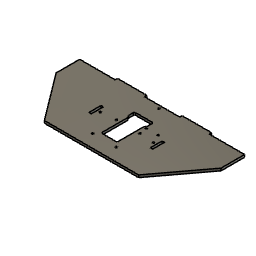
tablet_bottom_plate (Autodesk Fusion 360 design; units mm, degrees)
Autodesk Fusion 360 part; units mm, degrees
note: some values were not read from the file. Set by a fixed rule: the direction of a hole.
sketch "スケッチ1" plane through (0, 0, 0) normal (0, 1, 0) x (1, 0, 0)
  line L0 (140, -4) -> (140, -44)
  line L1 (140, -44) -> (80, -124)
  line L2 (80, -124) -> (-80, -124)
  line L3 (-80, -124) -> (-140, -44)
  line L4 (-140, -44) -> (-140, -4)
  line L5 (50, -54) -> (54, -54)
  line L6 (54, -54) -> (54, -74)
  line L7 (54, -74) -> (50, -74)
  line L8 (50, -74) -> (50, -54)
  line L9 (-54, -54) -> (-50, -54)
  line L10 (-50, -54) -> (-50, -74)
  line L11 (-50, -74) -> (-54, -74)
  line L12 (-54, -74) -> (-54, -54)
  line L13 (50, -64) -> (45, -64)
  line L14 (-50, -64) -> (-45, -64)
  line L15 (-140, -4) -> (-80, -4)
  line L16 (-80, -4) -> (-80, 0)
  line L17 (-80, 0) -> (-30, 0)
  line L18 (-30, 0) -> (-30, -4)
  line L19 (-30, -4) -> (30, -4)
  line L20 (30, -4) -> (30, 0)
  line L21 (30, 0) -> (80, 0)
  line L22 (80, 0) -> (80, -4)
  line L23 (80, -4) -> (140, -4)
  line L24 (0, -4) -> (0, -9)
  line L25 (-10, -96) -> (10, -96)
  line L26 (10, -96) -> (10, -92)
  line L27 (10, -92) -> (-10, -92)
  line L28 (-10, -92) -> (-10, -96)
  line L29 (-60, -78.5) -> (60, -78.5)
  line L30 (-75, -96) -> (-55, -96)
  line L31 (-55, -96) -> (-55, -104)
  line L32 (-55, -104) -> (-75, -104)
  line L33 (-75, -104) -> (-75, -96)
  line L34 (-20, -62) -> (20, -62)
  line L35 (20, -62) -> (20, -102)
  line L36 (20, -102) -> (-20, -102)
  line L37 (-20, -102) -> (-20, -62)
  line L38 (-13.5, -47) -> (13.5, -47)
  line L39 (13.5, -47) -> (13.5, -94)
  line L40 (13.5, -94) -> (-13.5, -94)
  line L41 (-13.5, -94) -> (-13.5, -47)
  line L42 (-16, -35) -> (16, -35)
  line L43 (16, -35) -> (16, -47)
  line L44 (16, -47) -> (-16, -47)
  line L45 (-16, -47) -> (-16, -35)
  point P0 (0, -124)
  point P1 (0, -4)
  point P2 (0, -96)
  point P3 (0, -78.5)
  point P4 (0, -62)
  point P5 (0, -47)
  dimension "d1" = 280
  dimension "d2" = 40
  dimension "d3" = 80
  dimension "d4" = 160
  dimension "d8" = 20
  dimension "d9" = 4
  dimension "d10" = 50
  dimension "d11" = 50
  dimension "d12" = 5
  dimension "d13" = 5
  dimension "d17" = 4
  dimension "d18" = 60
  dimension "d19" = 60
  dimension "d20" = 60
  dimension "d22" = 50
  dimension "d23" = 5
  dimension "d24" = 28
  dimension "d25" = 4
  dimension "d26" = 20
  dimension "d27" = 13.5
  dimension "d28" = 120
  dimension "d29" = 20
  dimension "d30" = 8
  dimension "d31" = 45
  dimension "d32" = 40
  dimension "d33" = 40
  dimension "d34" = 62
  dimension "d35" = 27
  dimension "d36" = 15
  dimension "d37" = 32
  dimension "d38" = 12
  dimension "d39" = 32
  constraint vertical L4
  constraint equal L1 L3
  constraint equal L0 L4
  constraint horizontal L5
  constraint vertical L6
  constraint horizontal L7
  constraint vertical L8
  constraint horizontal L9
  constraint vertical L10
  constraint horizontal L11
  constraint vertical L12
  constraint collinear L5 L9
  constraint collinear L7 L11
  constraint equal L5 L9
  constraint midpoint L8 L13.start
  constraint perpendicular L8 L13
  constraint midpoint L10 L14.start
  constraint perpendicular L10 L14
  constraint horizontal L2
  constraint vertical L0
  constraint horizontal L0.end L3.end
  constraint perpendicular L4 L15
  constraint perpendicular L15 L16
  constraint perpendicular L16 L17
  constraint perpendicular L15 L18
  constraint perpendicular L18 L19
  constraint perpendicular L19 L20
  constraint perpendicular L20 L21
  constraint perpendicular L19 L22
  constraint perpendicular L22 L23
  constraint coincident L0.start L23.end
  constraint midpoint L2 P0
  constraint midpoint L19 P1
  constraint vertical origin P1
  constraint vertical P0 P1
  constraint collinear L19 L23
  constraint collinear L17 L21
  constraint horizontal origin L20.end
  constraint coincident P1 L24.start
  constraint perpendicular L19 L24
  constraint horizontal L25
  constraint vertical L26
  constraint horizontal L27
  constraint vertical L28
  constraint midpoint L25 P2
  constraint vertical P0 P2
  constraint parallel L27 L29
  constraint midpoint L29 P3
  constraint vertical P0 P3
  constraint horizontal L30
  constraint vertical L31
  constraint horizontal L32
  constraint vertical L33
  constraint collinear L25 L30
  constraint horizontal L34
  constraint vertical L35
  constraint horizontal L36
  constraint vertical L37
  constraint midpoint L34 P4
  constraint vertical origin P4
  constraint horizontal L38
  constraint vertical L39
  constraint horizontal L40
  constraint vertical L41
  constraint midpoint L38 P5
  constraint vertical origin P5
  constraint horizontal L42
  constraint vertical L43
  constraint horizontal L44
  constraint vertical L45
  constraint midpoint P5 L44
  measures "d1" distance of L0.start L4.end
  measures "d2" distance of L0.start L0.end
  measures "d3" vertical distance of L0.end L1.end
  measures "d4" distance of L1.end L2.end
  measures "d8" distance of L5.end L6.end
  measures "d9" distance of L6.end L7.end
  measures "d10" distance of origin L8
  measures "d11" distance of origin L10
  measures "d12" distance of L14.start L14.end
  measures "d13" distance of L13.start L13.end
  measures "d17" distance of L15.end L16.end
  measures "d18" distance of L18.end L19.end
  measures "d19" distance of L4.end L15.end
  measures "d20" distance of L22.end L0.start
  measures "d22" distance of L5 L19
  measures "d23" distance of P1 L24.end
  measures "d24" distance of L2 L25
  measures "d25" distance of L25.end L26.end
  measures "d26" distance of L26.end L27.end
  measures "d27" distance of L27 L29
  measures "d28" distance of L29.start L29.end
  measures "d29" distance of L30.start L30.end
  measures "d30" distance of L30.start L32.end
  measures "d31" distance of L25.start L31
  measures "d32" distance of L34.start L34.end
  measures "d33" distance of L34.end L35.end
  measures "d34" distance of origin L34
  measures "d35" distance of L38.start L38.end
  measures "d36" distance of L34 L38
  measures "d37" distance of L34 L40
  measures "d38" distance of L42 L44
  measures "d39" distance of L42.start L42.end
extrude "押し出し1" add sketch "スケッチ1" along normal blind 4 contours L0 L1 L2 L3 L4 L15 L16 L17 L18 L19 L20 L21 L22 L23 | L25 L26 L28 L40 | L25 L26 L28 L29 L35 L36 L37 L39 L40 L41 | L29 L34 L37 L41 | L29 L34 L35 L39 | L30 L31 L32 L33
hole "穴1" at (-45, 0, 64) at (45, 0, 64) at (0, 0, 9) at (-20, 0, 102) at (-20, 0, 62) at (20, 0, 62) at (20, 0, 102) direction (0, 1, 0) diameter 3.2 depth 4 tip angle 118
fillet "フィレット1" radius 2 8 edges at (-16, 2, 35) (16, 2, 35) (16, 2, 47) (13.5, 2, 47) (-16, 2, 47) (-13.5, 2, 47) (-13.5, 2, 94) (13.5, 2, 94)
sketch "スケッチ2" plane through (0, 4, 0) normal (0, 1, 0) x (-1, 0, 0)
  circle A0 centre (-20, 62) radius 1.6
  circle A1 centre (20, 102) radius 1.6
  circle A2 centre (-45, 64) radius 1.6
  circle A3 centre (45, 64) radius 1.6
  circle A4 centre (0, 9) radius 1.6
  circle A5 centre (20, 62) radius 1.6
  circle A6 centre (-20, 102) radius 1.6
  line L0 (-54, 74) -> (-50, 74)
  line L1 (-50, 74) -> (-50, 54)
  line L2 (-50, 54) -> (-54, 54)
  line L3 (-54, 54) -> (-54, 74)
  line L4 (50, 74) -> (54, 74)
  line L5 (54, 74) -> (54, 54)
  line L6 (54, 54) -> (50, 54)
  line L7 (50, 54) -> (50, 74)
  arc A7 (13.5, 48.7081) -> (14.75, 46.854) centre (15.5, 48.7081) ccw
  arc A8 (16, 45) -> (14.75, 46.854) centre (14, 45) ccw
  line L8 (16, 45) -> (16, 37)
  arc A9 (14, 35) -> (16, 37) centre (14, 37) ccw
  line L9 (14, 35) -> (-14, 35)
  arc A10 (-16, 37) -> (-14, 35) centre (-14, 37) ccw
  line L10 (-16, 37) -> (-16, 45)
  arc A11 (-14.75, 46.854) -> (-16, 45) centre (-14, 45) ccw
  arc A12 (-14.75, 46.854) -> (-13.5, 48.7081) centre (-15.5, 48.7081) ccw
  line L11 (-13.5, 48.7081) -> (-13.5, 92)
  arc A13 (-11.5, 94) -> (-13.5, 92) centre (-11.5, 92) ccw
  line L12 (-11.5, 94) -> (11.5, 94)
  arc A14 (13.5, 92) -> (11.5, 94) centre (11.5, 92) ccw
  line L13 (13.5, 92) -> (13.5, 48.7081)
  line L14 (-80, 4) -> (-80, 0)
  line L15 (-80, 0) -> (-30, 0)
  line L16 (-30, 0) -> (-30, 4)
  line L17 (-30, 4) -> (30, 4)
  line L18 (30, 4) -> (30, 0)
  line L19 (30, 0) -> (80, 0)
  line L20 (80, 0) -> (80, 4)
  line L21 (80, 4) -> (140, 4)
  line L22 (140, 4) -> (140, 44)
  line L23 (140, 44) -> (80, 124)
  line L24 (80, 124) -> (-80, 124)
  line L25 (-80, 124) -> (-140, 44)
  line L26 (-140, 44) -> (-140, 4)
  line L27 (-140, 4) -> (-80, 4)
  line L28 (-18, 49) -> (-38, 49)
  dimension "d42" = 20
  dimension "d43" = 45
  dimension "d44" = 18
  constraint horizontal L28
  measures "d42" distance of L28.start L28.end
  measures "d43" distance of L17 L28
  measures "d44" horizontal distance of origin L28.start
hole "穴2" at (18, 4, 49) at (38, 4, 49) direction (0, -1, 0) diameter 3 end through all
